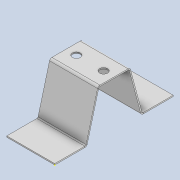
# Autodesk Inventor part: placa tierra
Saved by Autodesk Inventor 2021 (Build 250183000, 183)
## iProperties
Created: 2021-06-19
Part Number: placa tierra
Material: Genérico
Document SubType Name: Chapa
Designer: Admin
Density: 1 g/cm^3
Sheet Metal Rule: Por defecto_mm
Appearance: Valor por defecto
Author: Admin
Autodesk Inventor part; units mm, degrees
ref_plane "YZ Plane" through (0, 0, 0) normal (1, 0, 0) x (0, 1, 0)
ref_plane "XZ Plane" through (0, 0, 0) normal (0, 1, 0) x (-1, 0, 0)
ref_plane "XY Plane" through (0, 0, 0) normal (0, 0, 1) x (1, 0, 0)
sketch "Boceto1" plane through (0, 0, 0) normal (0, 1, 0) x (-1, 0, 0)
  point P0 (0, 0)
sketch "Boceto2" plane through (0, 0, 0) normal (0, 1, 0) x (-1, 0, 0)
  line L0 (0, 0) -> (30, 0)
  line L1 (30, 0) -> (30, -20)
  line L2 (30, -20) -> (0, -20)
  line L3 (0, -20) -> (0, 0)
  dimension "d0" = 30
  dimension "d1" = 20
  measures "d0" distance of L1.end L2.end
  measures "d1" distance of L0.end L1.end
extrude "Placa1" add sketch "Boceto2" along normal blind 0.76
sketch "Boceto3" plane through (0, 0.1967, -19.2659) normal (0, -0.258819, -0.9659258) x (-1, 0, 0)
  line L0 (30, 0) -> (0, 0)
  line L1 (0, 0) -> (0, -30)
  line L2 (0, -30) -> (30, -30)
  line L3 (30, -30) -> (30, 0)
  constraints: 6 end point, 1 horizontal, 1 perpendicular, 1 vertical
edge flange "Pestaña1" height 30 angle -75 thickness 0.76 bend radius 0.76 thickness toward (0, -0.258819, -0.9659258) relief straight relief width 0.76 relief depth 0.38 edges at (-15, 0, -20) wall of the first edge with corners at (-30, 0.1967, -19.2659) (0, 0.1967, -19.2659) (0, 29.1745, -27.0305) (-30, 29.1745, -27.0305)
bend "Doblez1"
corner "Esquina1"
sketch "Boceto4" plane through (-30, 28.4145, -27.0305) normal (0, 1, 0) x (-1, 0, 0)
  line L0 (-30, 0) -> (0, 0)
  line L1 (0, 0) -> (0, 20)
  line L2 (0, 20) -> (-30, 20)
  line L3 (-30, 20) -> (-30, 0)
  constraints: 6 end point, 1 horizontal, 1 perpendicular, 1 vertical
edge flange "Pestaña2" height 20 angle -75 thickness 0.76 bend radius 0.76 thickness toward (0, 1, 0) relief straight relief width 0.76 relief depth 0.38 edges at (-15, 29.1745, -27.0305) wall of the first edge with corners at (0, 28.4145, -27.0305) (-30, 28.4145, -27.0305) (-30, 28.4145, -47.0305) (0, 28.4145, -47.0305)
bend "Doblez2"
corner "Esquina2"
sketch "Boceto5" plane through (-30, 28.9778, -46.2964) normal (0, 0.258819, -0.9659258) x (1, 0, 0)
  line L0 (30, 0) -> (0, 0)
  line L1 (0, 0) -> (0, -30)
  line L2 (0, -30) -> (30, -30)
  line L3 (30, -30) -> (30, 0)
  constraints: 6 end point, 1 horizontal, 1 perpendicular, 1 vertical
edge flange "Pestaña3" height 30 angle -75 thickness 0.76 bend radius 0.76 thickness toward (0, 0.258819, -0.9659258) relief straight relief width 0.76 relief depth 0.38 edges at (-15, 29.1745, -47.0305) wall of the first edge with corners at (0, 28.9778, -46.2964) (-30, 28.9778, -46.2964) (-30, 0, -54.0609) (0, 0, -54.0609)
bend "Doblez3"
corner "Esquina3"
sketch "Boceto6" plane through (0, 0.76, -54.0609) normal (0, -1, 0) x (1, 0, 0)
  line L0 (-30, 0) -> (0, 0)
  line L1 (0, 0) -> (0, 20)
  line L2 (0, 20) -> (-30, 20)
  line L3 (-30, 20) -> (-30, 0)
  constraints: 6 end point, 1 horizontal, 1 perpendicular, 1 vertical
edge flange "Pestaña4" height 20 angle -75 thickness 0.76 bend radius 0.76 thickness toward (0, -1, 0) relief straight relief width 0.76 relief depth 0.38 edges at (-15, 0, -54.0609) wall of the first edge with corners at (-30, 0.76, -54.0609) (0, 0.76, -54.0609) (0, 0.76, -74.0609) (-30, 0.76, -74.0609)
bend "Doblez4"
corner "Esquina4"
sketch "Boceto7" plane through (-30, 29.1745, -28.1968) normal (0, 1, 0) x (1, 0, 0)
  circle A0 centre (6.5, 8.8337) radius 2.5
  circle A1 centre (23.5, 8.8337) radius 2.5
  line L0 (0, 0) -> (0, 17.6673) projected
  line L1 (30, 0) -> (30, 17.6673) projected
  point P0 (30, -28.1968)
  dimension "d43" = 5
  dimension "d44" = 5
  dimension "d45" = 6.5
  dimension "d46" = 6.5
  constraints: 2 centre point
  measures "d43" diameter of A0
  measures "d44" diameter of A1
  measures "d45" distance from line of L0 A0.centre
  measures "d46" distance from line of A1.centre L1
extrude "Extrusión1" cut sketch "Boceto7" against normal through all
equation "\"d46\" = d45"
equation "\"d2\" = Grosor"
equation "\"d3\" = Anchura_desahogo_plegado"
equation "\"d4\" = Profundidad_desahogo_plegado"
equation "\"d5\" = Remanente_mínimo"
equation "\"d6\" = Radiodetransición"
equation "\"d9\" = Radio_pliegue"
equation "\"d10\" = Tamaño_destalonado"
equation "\"d11\" = TamañoSeparación"
equation "\"d12\" = Tamaño_de_radio_de_Jacobi"
equation "\"d13\" = Anchura_desahogo_plegado"
equation "\"d14\" = Profundidad_desahogo_plegado"
equation "\"d15\" = Remanente_mínimo"
equation "\"d16\" = Radiodetransición"
equation "\"d19\" = Radio_pliegue"
equation "\"d20\" = Tamaño_destalonado"
equation "\"d21\" = TamañoSeparación"
equation "\"d22\" = Tamaño_de_radio_de_Jacobi"
equation "\"d23\" = Anchura_desahogo_plegado"
equation "\"d24\" = Profundidad_desahogo_plegado"
equation "\"d25\" = Remanente_mínimo"
equation "\"d26\" = Radiodetransición"
equation "\"d29\" = Radio_pliegue"
equation "\"d30\" = Tamaño_destalonado"
equation "\"d31\" = TamañoSeparación"
equation "\"d32\" = Tamaño_de_radio_de_Jacobi"
equation "\"d33\" = Anchura_desahogo_plegado"
equation "\"d34\" = Profundidad_desahogo_plegado"
equation "\"d35\" = Remanente_mínimo"
equation "\"d36\" = Radiodetransición"
equation "\"d39\" = Radio_pliegue"
equation "\"d40\" = Tamaño_destalonado"
equation "\"d41\" = TamañoSeparación"
equation "\"d42\" = Tamaño_de_radio_de_Jacobi"
equation "\"Radio_pliegue\" = Grosor"
equation "\"Anchura_desahogo_plegado\" = Grosor"
equation "\"Profundidad_desahogo_plegado\" = 0.5 * Grosor"
equation "\"Tamaño_destalonado\" = 4 * Grosor"
equation "\"Remanente_mínimo\" = 2 * Grosor"
equation "\"Radiodetransición\" = Radio_pliegue"
equation "\"Tamaño_de_radio_de_Jacobi\" = Radio_pliegue"
equation "\"TamañoSeparación\" = Grosor"
equation "\"Grosor\" = 0.76"
